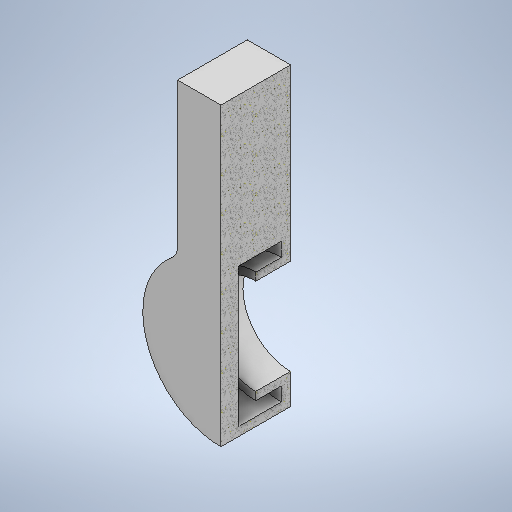
# Autodesk Inventor part: alternativeJoint
Saved by Autodesk Inventor 2025.1 (Build 291241000, 241)
## iProperties
Created: 2024-11-06
Part Number: alternativeJoint
Material: Generisch
Document SubType Name: Modeling
Designer: ZOMBULLI
Density: 1 g/cm^3
Appearance: Vorgabe
Author: ZOMBULLI
Autodesk Inventor part; units mm, degrees
ref_plane "YZ Plane" through (0, 0, 0) normal (1, 0, 0) x (0, 1, 0)
ref_plane "XZ Plane" through (0, 0, 0) normal (0, 1, 0) x (-1, 0, 0)
ref_plane "XY Plane" through (0, 0, 0) normal (0, 0, 1) x (1, 0, 0)
sketch "Skizze1" plane through (0, 0, 0) normal (0, 1, 0) x (-1, 0, 0)
  line L0 (5, 25) -> (-5, 25)
  line L1 (-5, 25) -> (-5, 9.3808)
  line L2 (5, 8.4853) -> (5, 25)
  arc A0 (-6.2308, 6.4944) -> (5.7273, 6.9425) centre (0, 0) ccw
  arc A1 (5, 8.4853) -> (5.7273, 6.9425) centre (7, 8.4853) ccw
  arc A2 (-6.2308, 6.4944) -> (-5, 9.3808) centre (-9, 9.3808) ccw
  line L3 (0, -16.1968) -> (0, 31.8661) projected
  point P0 (0, 0)
  point P1 (-5, 7.4833)
  point P2 (5, 7.4833)
  dimension "d2" = 18
  dimension "d3" = 5
  dimension "d4" = 2
  dimension "d5" = 4
  dimension "d8" = 10
  dimension "d9" = 5
  dimension "d10" = 0
  dimension "d11" = 25
  constraints: 8 point on circle, 6 end point, 4 tangent, 3 centre point, 2 point on line, 1 horizontal, 1 parallel, 1 perpendicular
  measures "d2" diameter of A0
  measures "d3" distance from line of A0.centre L2
  measures "d4" radius of A1
  measures "d5" radius of A2
  measures "d8" distance between parallel lines of L1 L2
  measures "d9" distance between parallel lines of L3 L2
  measures "d10" distance of A0.centre point (0, 0)
  measures "d11" distance from line of point (0, 0) L0
extrude "Extrusion1" add sketch "Skizze1" along normal blind 8
sketch "Skizze3" plane through (0, 8, 0) normal (0, 1, 0) x (1, 0, 0)
  circle A0 centre (0, 0) radius 5.5
  dimension "d12" = 11
  constraints: 1 centre point, 1 coincident
  measures "d12" diameter of A0
extrude "Extrusion2" cut sketch "Skizze3" against normal blind 6
sketch "Skizze5" plane through (0, 0, 0) normal (1, 0, 0) x (0, 1, 0)
  line L0 (4, 0) -> (2, 0)
  line L1 (2, 0) -> (2, -8)
  line L2 (4, -6.4) -> (4, 0)
  line L3 (2, 5.5) -> (2, -5.5) projected
  line L4 (4, -6.4) -> (6.9352, -6.4)
  line L5 (6.9352, -6.4) -> (6.9352, -8)
  line L6 (6.9352, -8) -> (2, -8)
  line L7 (-1.387, 0) -> (8.3222, 0) projected
  point P0 (0, 0)
  point P1 (3, 0)
  point P2 (5.4676, -6.4)
  dimension "d21" = 0
  dimension "d22" = 2
  dimension "d26" = 8
  dimension "d27" = 6.4
  constraints: 12 end point, 3 horizontal, 2 midpoint, 2 perpendicular, 1 parallel
  measures "d21" distance between parallel lines of L3 L1
  measures "d22" distance of L0.start L0.end
  measures "d26" distance from line of L5.end L7
  measures "d27" distance from line of point (5.468, -6.4) L7
revolve "Umdrehung1" cut sketch "Skizze5" angle 360 about axis through (0, 4, 0) along (0, -1, 0)
